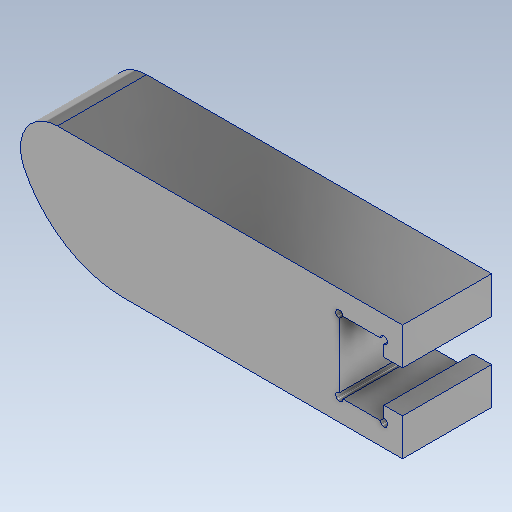
# Autodesk Inventor part: Finray_9_Kerbe_10deg_anschluss_erweitert_9_75 Nut
Saved by Autodesk Inventor 2025.2 (Build 292293000, 293)
## iProperties
Created: 2022-02-28
Part Number: Finray_9_Kerbe_10deg_anschluss_erweitert_9_75 Nut
Material: Generic
Document SubType Name: Modeling
Designer: richa
Density: 1 g/cm^3
Appearance: Aluminum - Flat
Author: richa
## iProperties of the stored document Maria_Greifer_3D-Druck.ipt
Created: 2024-11-10
Part Number: Maria_Greifer_3D-Druck
Material: Generisch
Document SubType Name: Modeling
Designer: maria
Density: 1 g/cm^3
Appearance: Vorgabe
Author: maria
Autodesk Inventor part; units mm, degrees
ref_plane "YZ Plane" through (0, 0, 0) normal (1, 0, 0) x (0, 1, 0)
ref_plane "XZ Plane" through (0, 0, 0) normal (0, 1, 0) x (-1, 0, 0)
ref_plane "XY Plane" through (0, 0, 0) normal (0, 0, 1) x (1, 0, 0)
sketch "Sketch5" plane through (0, 0, 0) normal (0, 0, 1) x (1, 0, 0)
  line L0 (52.5, -15.6) -> (52.5, -10.6)
  line L1 (52.5, -10.6) -> (50, -10.6)
  line L2 (50, -10.6) -> (50, -12.625)
  line L3 (44, -12.625) -> (44, -2.975)
  line L4 (50, -2.975) -> (50, -5)
  line L5 (50, -5) -> (52.5, -5)
  line L6 (52.5, -5) -> (52.5, 0)
  line L7 (52.5, 0) -> (7.8, 0)
  line L8 (44, -2.975) -> (50, -2.975)
  line L9 (44, -12.625) -> (50, -12.625)
  line L10 (52.5, -15.6) -> (7.8, -15.6)
  line L11 (7.8, -15.6) -> (0, -15.6)
  line L12 (0, -15.6) -> (0, 0)
  line L13 (0, 0) -> (7.8, 0)
  point P0 (7.8, 0)
  dimension "d41" = 6
  dimension "d48" = 44
  dimension "d50" = 2.5
  dimension "d63" = 44.7
  dimension "d71" = 0
  dimension "d87" = 5.6
  dimension "d88" = 9.65
  dimension "d97" = 15.6
  constraints: 28 end point, 8 perpendicular, 4 collinear, 3 parallel, 2 horizontal, 1 vertical
  measures "d41" distance between parallel lines of L2 L3
  measures "d48" distance from line of L3 L12.end
  measures "d50" distance of L4.end L5.end
  measures "d63" distance of L0.start L10.end
  measures "d71" distance from line of L12.end L7
  measures "d87" distance from line of L0.end L5
  measures "d88" distance of L3.start L3.end
  measures "d97" distance of L11.end L12.end
extrude "Extrusion2" add sketch "Sketch5" along normal blind 12
fillet "Fillet2" radius 15 1 edges at (0, -15.6, 6)
sketch "Sketch11" plane through (0, 0, 12) normal (0, 0, 1) x (1, 0, 0)
  line L0 (44, -2.975) -> (50, -2.975) projected
  circle A0 centre (44, -2.975) radius 0.5
  line L1 (44, -12.625) -> (44, -2.975) projected
  circle A1 centre (44, -12.625) radius 0.5
  line L2 (50, -12.625) -> (44, -12.625) projected
  circle A2 centre (50, -12.625) radius 0.5
  line L3 (50, -2.975) -> (50, -5) projected
  circle A3 centre (50, -2.975) radius 0.5
  point P0 (0, 0)
  dimension "d99" = 1
  dimension "d100" = 1
  dimension "d101" = 1
  dimension "d102" = 1
  constraints: 4 centre point, 1 coincident
  measures "d99" diameter of A0
  measures "d100" diameter of A1
  measures "d101" diameter of A2
  measures "d102" diameter of A3
extrude "Extrusion7" cut sketch "Sketch11" against normal through all
fillet "Rundung3" radius 5 1 edges at (0, 0, 6)
equation "\"l1\" = 8"
body "Solid2"
